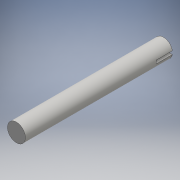
# Autodesk Inventor part: Solenoid Interior
Saved by Autodesk Inventor 2016 (Build 200138000, 138)
## iProperties
Created: 2016-05-08
Part Number: Solenoid Interior
Material: Generic
Document SubType Name: Modeling
Designer: Kenneth Daniel
Density: 1 g/cm^3
Appearance: Default
Author: Kenneth Daniel
Autodesk Inventor part; units mm, degrees
ref_plane "YZ Plane" through (0, 0, 0) normal (1, 0, 0) x (0, 1, 0)
ref_plane "XZ Plane" through (0, 0, 0) normal (0, 1, 0) x (-1, 0, 0)
ref_plane "XY Plane" through (0, 0, 0) normal (0, 0, 1) x (1, 0, 0)
sketch "Sketch1" plane through (0, 0, 0) normal (0, 1, 0) x (-1, 0, 0)
  circle A0 centre (0, 0) radius 2.75
  dimension "d0" = 5.5
  constraints: 1 centre point, 1 coincident
  measures "d0" diameter of A0
extrude "Extrusion1" add sketch "Sketch1" along normal blind 45
sketch "Sketch2" plane through (0, 45, 0) normal (0, 1, 0) x (1, 0, 0)
  line L0 (3.6897, -0.5) -> (3.6897, 0.5)
  line L1 (3.6897, 0.5) -> (-3.6897, 0.5)
  line L2 (-3.6897, 0.5) -> (-3.6897, -0.5)
  line L3 (-3.6897, -0.5) -> (3.6897, -0.5)
  line L4 (3.6897, -0.5) -> (-3.6897, 0.5) construction
  line L5 (3.6897, 0.5) -> (-3.6897, -0.5) construction
  point P0 (0, 0)
  dimension "d3" = 1
  constraints: 12 end point, 2 midpoint, 2 parallel, 1 perpendicular, 1 vertical
  measures "d3" distance of L0.start L0.end
extrude "Extrusion2" cut sketch "Sketch2" against normal blind 5
body "Solid1"
